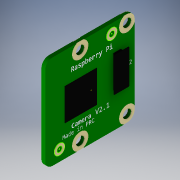
# Autodesk Inventor part: PicameraPCB
Saved by Autodesk Inventor 2022 (Build 260153000, 153)
## iProperties
Created: 2018-02-01
Part Number: PicameraPCB
Material: Genérico
Document SubType Name: Modeling
Designer: RafaX
Density: 1 g/cm^3
Appearance: Valor por defecto
Author: RafaX
Autodesk Inventor part; units mm, degrees
(part 1 of 2)
sketch "Boceto1" plane through (0, 0, 0) normal (0, 0, 1) x (1, 0, 0)
  line L0 (-9.7561, 12.3858) -> (10.1059, 12.3858)
  line L1 (12.1059, 10.3858) -> (12.1059, -10.6142)
  line L2 (10.1059, -12.6142) -> (-9.7561, -12.6142)
  line L3 (-11.7561, -10.6142) -> (-11.7561, 10.3858)
  arc A0 (-11.7561, -10.6142) -> (-9.7561, -12.6142) centre (-9.7561, -10.6142) ccw
  arc A1 (10.1059, -12.6142) -> (12.1059, -10.6142) centre (10.1059, -10.6142) ccw
  arc A2 (12.1059, 10.3858) -> (10.1059, 12.3858) centre (10.1059, 10.3858) ccw
  arc A3 (-9.7561, 12.3858) -> (-11.7561, 10.3858) centre (-9.7561, 10.3858) ccw
  point P0 (0, 0)
  point P1 (-11.7561, 12.3858)
  point P2 (12.1059, -12.6142)
  point P3 (12.1059, 12.3858)
  point P4 (-11.7561, -12.6142)
  point P5 (-9.7561, -10.6142)
  point P6 (2.7439, -10.6142)
  point P7 (-9.7561, 10.3858)
  point P8 (2.7439, 10.3858)
  dimension "d0" = 23.862
  dimension "d1" = 25
  dimension "d7" = 2
  dimension "d8" = 2
  dimension "d11" = 12.5
  dimension "d14" = 21
  dimension "d26" = 2
  constraints: 8 end point, 8 point on circle, 8 point on line, 8 tangent, 4 centre point, 3 equal radius, 2 horizontal, 2 parallel, 1 perpendicular, 1 vertical, 3 other
  measures "d0" distance of point (-11.756, 12.386) point (12.106, 12.386)
  measures "d1" distance of point (12.106, 12.386) point (12.106, -12.614)
  measures "d7" distance from line of L2 point (-9.756, -10.614)
  measures "d8" distance from line of L3 point (-9.756, -10.614)
  measures "d11" distance of point (-9.756, -10.614) point (2.744, -10.614)
  measures "d14" distance of point (-9.756, -10.614) point (-9.756, 10.386)
  measures "d26" radius of A0
extrude "PCB_EXT" add sketch "Boceto1" along normal blind 1
hole "PADS_PCB_DRILL" at (-9.7561, -10.6142, 0) at (2.7439, -10.6142, 0) at (-9.7561, 10.3858, 0) at (2.7439, 10.3858, 0) direction (0, 0, 1) diameter 2.2 end through all counterbore diameter 4.4 counterbore depth 0.12
sketch "Boceto2" plane through (0, 0, 1) normal (0, 0, 1) x (1, 0, 0)
  circle A0 centre (2.7468, 10.3904) radius 2.2
  circle A1 centre (2.7468, -10.6245) radius 2.2
  circle A2 centre (-9.7649, 10.3904) radius 2.2
  circle A3 centre (-9.7649, -10.6245) radius 2.2
  point P0 (0, 0)
  point P1 (2.7439, 10.3858)
  dimension "d27" = 4.4
  dimension "d28" = 4.4
  dimension "d29" = 4.4
  dimension "d30" = 4.4
  constraints: 4 centre point
  measures "d27" diameter of A0
  measures "d28" diameter of A1
  measures "d29" diameter of A2
  measures "d30" diameter of A3
extrude "PADS_PCB_DRILL_EXT" cut sketch "Boceto2" against normal blind 0.13
sketch "FOTO" plane through (0, 0, 1) normal (0, 0, 1) x (1, 0, 0)
  line L0 (-11.6696, 12.3223) -> (12.1528, 12.3223) construction
  line L1 (12.1528, 12.3223) -> (12.1528, -12.4777) construction
  line L2 (12.1528, -12.4777) -> (-11.6696, -12.4777) construction
  line L3 (-11.6696, -12.4777) -> (-11.6696, 12.3223) construction
  point P0 (0, 0)
  dimension "d57" = 24.8
  constraints: 2 other
  measures "d57" distance of L0.end L1.end
ref_plane "SUPERIOR_PADS" through (6.4264, 12.3858, 0.87) normal (0, 0, 1) x (1, 0, 0)
sketch "Boceto4" plane through (6.4264, 12.3858, 0.87) normal (0, 0, 1) x (1, 0, 0)
  arc A0 (-15.2525, -25) -> (-18.1824, -22.0747) centre (-16.1913, -23.0104) ccw projected
  arc A1 (-18.1824, -2.9311) -> (-15.2649, 0) centre (-16.1913, -1.9954) ccw projected
  arc A2 (-4.606, 0) -> (-2.7532, 0) centre (-3.6796, -1.9954) ccw projected
  circle A3 centre (-16.1824, -23) radius 1.1 projected
  circle A4 centre (-3.6824, -23) radius 1.1 projected
  line L0 (-18.1824, -2.9311) -> (-18.1824, -2) projected
  arc A5 (-16.1824, 0) -> (-18.1824, -2) centre (-16.1824, -2) ccw projected
  line L1 (-16.1824, 0) -> (-15.2649, 0) projected
  arc A6 (-16.1824, 0) -> (-18.1824, -2) centre (-16.1824, -2) ccw projected
  line L2 (-18.1824, -2.9311) -> (-18.1824, -2) projected
  arc A7 (-18.1824, -2.9311) -> (-15.2649, 0) centre (-16.1913, -1.9954) ccw projected
  circle A8 centre (-16.1824, -2) radius 1.1 projected
  line L3 (-4.606, 0) -> (-2.7532, 0) projected
  line L4 (-2.7408, -25) -> (-4.6184, -25) projected
  line L5 (-15.2525, -25) -> (-16.1824, -25) projected
  arc A9 (-18.1824, -23) -> (-16.1824, -25) centre (-16.1824, -23) ccw projected
  line L6 (-18.1824, -23) -> (-18.1824, -22.0747) projected
  circle A10 centre (-3.6824, -2) radius 1.1 projected
  arc A11 (-2.7408, -25) -> (-4.6184, -25) centre (-3.6796, -23.0104) ccw projected
  point P0 (-6.4264, -12.3858)
extrude "PADS_GOLDEN_UPPER_EXT" add sketch "Boceto4" along normal blind 0.07 separate body
ref_plane "INFERIOR_PADS" through (-3.5061, -12.6142, 0.12) normal (0, 0, -1) x (1, 0, 0)
sketch "Boceto5" plane through (-3.5061, -12.6142, 0.12) normal (0, 0, -1) x (1, 0, 0)
  line L0 (-6.25, 0) -> (-5.3335, 0) projected
  arc A0 (-6.25, 0) -> (-8.25, -2) centre (-6.25, -2) ccw projected
  line L1 (-8.25, -2.9165) -> (-8.25, -2) projected
  arc A1 (-8.25, -2.9165) -> (-5.3335, 0) centre (-6.25, -2) ccw projected
  circle A2 centre (-6.25, -2) radius 1.1 projected
  line L2 (5.3335, 0) -> (7.1665, 0) projected
  arc A3 (5.3335, 0) -> (7.1665, 0) centre (6.25, -2) ccw projected
  circle A4 centre (6.25, -2) radius 1.1 projected
  line L3 (7.1665, -25) -> (5.3335, -25) projected
  arc A5 (7.1665, -25) -> (5.3335, -25) centre (6.25, -23) ccw projected
  circle A6 centre (6.25, -23) radius 1.1 projected
  circle A7 centre (-6.25, -23) radius 1.1 projected
  line L4 (-5.3335, -25) -> (-6.25, -25) projected
  arc A8 (-5.3335, -25) -> (-8.25, -22.0835) centre (-6.25, -23) ccw projected
  line L5 (-8.25, -23) -> (-8.25, -22.0835) projected
  arc A9 (-8.25, -23) -> (-6.25, -25) centre (-6.25, -23) ccw projected
  point P0 (3.5061, -12.6142)
extrude "PADS_GOLDEN_LOWER_EXT" add sketch "Boceto5" along normal blind 0.07 separate body
sketch "text_front" plane through (0, 0, 1) normal (0, 0, 1) x (1, 0, 0)
  line L0 (5.2786, -8.033) -> (-7.7766, -8.033) construction
  line L1 (-7.7766, -8.033) -> (-7.7766, -6.6244) construction
  line L2 (-7.7766, -6.6244) -> (5.2786, -6.6244) construction
  line L3 (5.2786, -6.6244) -> (5.2786, -8.033) construction
  line L4 (-9.4094, -1.7368) -> (-11.3059, -1.7368) construction
  line L5 (-11.3059, -1.7368) -> (-11.3059, -0.6092) construction
  line L6 (-11.3059, -0.6092) -> (-9.4094, -0.6092) construction
  line L7 (-9.4094, -0.6092) -> (-9.4094, -1.7368) construction
  line L8 (5.1279, 5.2449) -> (-0.7022, 5.2449) construction
  line L9 (-0.7022, 5.2449) -> (-0.7022, 6.6125) construction
  line L10 (-0.7022, 6.6125) -> (5.1279, 6.6125) construction
  line L11 (5.1279, 6.6125) -> (5.1279, 5.2449) construction
  line L12 (-1.2173, 5.1295) -> (-5.0625, 5.1295) construction
  line L13 (-5.0625, 5.1295) -> (-5.0625, 6.3628) construction
  line L14 (-5.0625, 6.3628) -> (-1.2173, 6.3628) construction
  line L15 (-1.2173, 6.3628) -> (-1.2173, 5.1295) construction
  line L16 (7.5273, 6.703) -> (-2.1657, 6.703) construction
  line L17 (-2.1657, 6.703) -> (-2.1657, 7.9173) construction
  line L18 (-2.1657, 7.9173) -> (7.5273, 7.9173) construction
  line L19 (7.5273, 7.9173) -> (7.5273, 6.703) construction
  line L20 (4.6281, -6.6975) -> (4.7797, -7.0835)
  spline S0 degree 2 poles (4.7797, -7.0835) (4.8012, -7.1384) (4.8775, -7.1943) (4.9302, -7.1943) knots 0 0 0 1 2 2 2
  line L21 (4.9302, -7.1943) -> (4.9689, -7.1943)
  line L22 (4.9689, -7.1943) -> (4.9689, -6.6975)
  line L23 (4.9689, -6.6975) -> (5.1721, -6.6975)
  line L24 (5.1721, -6.6975) -> (5.1721, -7.8975)
  line L25 (5.1721, -7.8975) -> (4.8571, -7.8975)
  spline S1 degree 2 poles (4.8571, -7.8975) (4.7678, -7.8975) (4.6227, -7.8642) (4.5205, -7.7846) (4.4646, -7.6577) (4.4646, -7.5663) knots 0 0 0 1 2 3 4 4 4
  spline S2 degree 2 poles (4.4646, -7.5663) (4.4646, -7.4997) (4.5001, -7.3975) (4.5625, -7.3233) (4.6496, -7.2771) (4.7001, -7.2674) knots 0 0 0 1 2 3 4 4 4
  spline S3 degree 2 poles (4.7001, -7.2674) (4.6603, -7.2588) (4.5947, -7.1771) (4.5614, -7.0997) knots 0 0 0 1 2 2 2
  line L26 (4.5614, -7.0997) -> (4.3893, -6.6975)
  line L27 (4.3893, -6.6975) -> (4.6281, -6.6975)
  spline S4 degree 2 poles (4.6786, -7.5438) (4.6786, -7.6319) (4.7786, -7.7093) (4.8797, -7.7093) knots 0 0 0 1 2 2 2
  line L28 (4.8797, -7.7093) -> (4.9689, -7.7093)
  line L29 (4.9689, -7.7093) -> (4.9689, -7.3706)
  line L30 (4.9689, -7.3706) -> (4.8861, -7.3706)
  spline S5 degree 2 poles (4.8861, -7.3706) (4.8388, -7.3706) (4.7625, -7.3921) (4.7076, -7.4362) (4.6786, -7.5018) (4.6786, -7.5438) knots 0 0 0 1 2 3 4 4 4
  line L31 (3.7076, -6.6975) -> (3.713, -6.8201)
  spline S6 degree 2 poles (3.713, -6.8201) (3.7388, -6.7889) (3.7969, -6.7362) (3.8657, -6.6975) (3.9474, -6.676) (3.9969, -6.676) knots 0 0 0 1 2 3 4 4 4
  spline S7 degree 2 poles (3.9969, -6.676) (4.0614, -6.676) (4.1582, -6.719) (4.2248, -6.7943) (4.2582, -6.9007) (4.2582, -6.9653) knots 0 0 0 1 2 3 4 4 4
  spline S8 degree 2 poles (4.2582, -6.9653) (4.2582, -7.0308) (4.2076, -7.1427) (4.1044, -7.2233) (3.9506, -7.2696) (3.8463, -7.2696) knots 0 0 0 1 2 3 4 4 4
  line L32 (3.8463, -7.2696) -> (3.7367, -7.2696)
  line L33 (3.7367, -7.2696) -> (3.7367, -7.3255)
  spline S9 degree 2 poles (3.7367, -7.3255) (3.7367, -7.361) (3.7549, -7.419) (3.7947, -7.4599) (3.8592, -7.4814) (3.9066, -7.4814) knots 0 0 0 1 2 3 4 4 4
  spline S10 degree 2 poles (3.9066, -7.4814) (3.9807, -7.4814) (4.1259, -7.4438) (4.1936, -7.4104) knots 0 0 0 1 2 2 2
  line L34 (4.1936, -7.4104) -> (4.1936, -7.5889)
  spline S11 degree 2 poles (4.1936, -7.5889) (4.1334, -7.6158) (3.9754, -7.6502) (3.8904, -7.6502) knots 0 0 0 1 2 2 2
  spline S12 degree 2 poles (3.8904, -7.6502) (3.7969, -7.6502) (3.6625, -7.6115) (3.5764, -7.5319) (3.5345, -7.4136) (3.5345, -7.3351) knots 0 0 0 1 2 3 4 4 4
  line L35 (3.5345, -7.3351) -> (3.5345, -6.6975)
  line L36 (3.5345, -6.6975) -> (3.7076, -6.6975)
  line L37 (3.7367, -7.1093) -> (3.8592, -7.1093)
  spline S13 degree 2 poles (3.8592, -7.1093) (3.9109, -7.1093) (3.9818, -7.0878) (4.0259, -7.0491) (4.0474, -6.9986) (4.0474, -6.9706) knots 0 0 0 1 2 3 4 4 4
  spline S14 degree 2 poles (4.0474, -6.9706) (4.0474, -6.9136) (3.9807, -6.8534) (3.9238, -6.8534) knots 0 0 0 1 2 2 2
  spline S15 degree 2 poles (3.9238, -6.8534) (3.8818, -6.8534) (3.7915, -6.9212) (3.7367, -6.9846) knots 0 0 0 1 2 2 2
  line L38 (3.7367, -6.9846) -> (3.7367, -7.1093)
  spline S16 degree 2 poles (2.6119, -6.9717) (2.6119, -6.8921) (2.6754, -6.7792) (2.7797, -6.7083) (2.913, -6.676) (2.9818, -6.676) knots 0 0 0 1 2 3 4 4 4
  spline S17 degree 2 poles (2.9818, -6.676) (3.0743, -6.676) (3.2238, -6.6954) (3.2893, -6.7136) knots 0 0 0 1 2 2 2
  line L39 (3.2893, -6.7136) -> (3.2893, -6.9158)
  spline S18 degree 2 poles (3.2893, -6.9158) (3.2119, -6.8803) (3.0571, -6.8481) (2.9893, -6.8481) knots 0 0 0 1 2 2 2
  spline S19 degree 2 poles (2.9893, -6.8481) (2.9098, -6.8481) (2.8313, -6.904) (2.8313, -6.9491) knots 0 0 0 1 2 2 2
  spline S20 degree 2 poles (2.8313, -6.9491) (2.8313, -6.9706) (2.8474, -7.005) (2.8936, -7.0373) (2.9754, -7.0717) (3.0431, -7.0921) knots 0 0 0 1 2 3 4 4 4
  spline S21 degree 2 poles (3.0431, -7.0921) (3.1044, -7.1115) (3.1979, -7.1599) (3.2592, -7.2265) (3.2893, -7.3136) (3.2893, -7.3728) knots 0 0 0 1 2 3 4 4 4
  spline S22 degree 2 poles (3.2893, -7.3728) (3.2893, -7.4298) (3.2431, -7.5308) (3.1517, -7.6061) (3.0141, -7.6502) (2.9227, -7.6502) knots 0 0 0 1 2 3 4 4 4
  spline S23 degree 2 poles (2.9227, -7.6502) (2.8431, -7.6502) (2.7216, -7.6319) (2.6743, -7.6212) knots 0 0 0 1 2 2 2
  line L40 (2.6743, -7.6212) -> (2.6743, -7.4384)
  spline S24 degree 2 poles (2.6743, -7.4384) (2.7463, -7.4642) (2.8721, -7.4857) (2.9345, -7.4857) knots 0 0 0 1 2 2 2
  spline S25 degree 2 poles (2.9345, -7.4857) (2.9969, -7.4857) (3.0711, -7.4362) (3.0711, -7.3921) knots 0 0 0 1 2 2 2
  spline S26 degree 2 poles (3.0711, -7.3921) (3.0711, -7.3706) (3.0571, -7.3373) (3.013, -7.3061) (2.9345, -7.2728) (2.87, -7.2524) knots 0 0 0 1 2 3 4 4 4
  spline S27 degree 2 poles (2.87, -7.2524) (2.7969, -7.2287) (2.6979, -7.1771) (2.6377, -7.1104) (2.6119, -7.0265) (2.6119, -6.9717) knots 0 0 0 1 2 3 4 4 4
  spline S28 degree 2 poles (1.6184, -7.1803) (1.6184, -7.0524) (1.684, -6.8642) (1.8001, -6.7405) (1.9592, -6.6814) (2.0517, -6.6814) knots 0 0 0 1 2 3 4 4 4
  spline S29 degree 2 poles (2.0517, -6.6814) (2.084, -6.6814) (2.1463, -6.69) (2.1721, -6.6975) knots 0 0 0 1 2 2 2
  line L41 (2.1721, -6.6975) -> (2.1721, -6.333)
  line L42 (2.1721, -6.333) -> (2.3732, -6.333)
  line L43 (2.3732, -6.333) -> (2.3732, -7.6308)
  line L44 (2.3732, -7.6308) -> (2.199, -7.6308)
  line L45 (2.199, -7.6308) -> (2.1947, -7.4932)
  spline S30 degree 2 poles (2.1947, -7.4932) (2.1689, -7.5287) (2.113, -7.5878) (2.0485, -7.6287) (1.9743, -7.6502) (1.9281, -7.6502) knots 0 0 0 1 2 3 4 4 4
  spline S31 degree 2 poles (1.9281, -7.6502) (1.8539, -7.6502) (1.7388, -7.5846) (1.6603, -7.462) (1.6184, -7.2889) (1.6184, -7.1803) knots 0 0 0 1 2 3 4 4 4
  spline S32 degree 2 poles (1.8302, -7.1717) (1.8302, -7.2481) (1.8496, -7.3567) (1.8872, -7.4265) (1.941, -7.4588) (1.9754, -7.4588) knots 0 0 0 1 2 3 4 4 4
  spline S33 degree 2 poles (1.9754, -7.4588) (2.027, -7.4588) (2.1195, -7.3674) (2.1721, -7.2878) knots 0 0 0 1 2 2 2
  line L46 (2.1721, -7.2878) -> (2.1721, -6.8803)
  spline S34 degree 2 poles (2.1721, -6.8803) (2.1485, -6.8706) (2.0775, -6.8577) (2.041, -6.8577) knots 0 0 0 1 2 2 2
  spline S35 degree 2 poles (2.041, -6.8577) (1.9936, -6.8577) (1.9152, -6.9018) (1.8592, -6.9825) (1.8302, -7.0986) (1.8302, -7.1717) knots 0 0 0 1 2 3 4 4 4
  spline S36 degree 2 poles (0.6883, -7.1803) (0.6883, -7.0524) (0.7539, -6.8642) (0.87, -6.7405) (1.0291, -6.6814) (1.1216, -6.6814) knots 0 0 0 1 2 3 4 4 4
  spline S37 degree 2 poles (1.1216, -6.6814) (1.2141, -6.6814) (1.3711, -6.7115) (1.4431, -6.7373) knots 0 0 0 1 2 2 2
  line L47 (1.4431, -6.7373) -> (1.4431, -7.9954)
  line L48 (1.4431, -7.9954) -> (1.242, -7.9954)
  line L49 (1.242, -7.9954) -> (1.242, -7.69)
  line L50 (1.242, -7.69) -> (1.2506, -7.5061)
  spline S38 degree 2 poles (1.2506, -7.5061) (1.2044, -7.5717) (1.0829, -7.6502) (0.9979, -7.6502) knots 0 0 0 1 2 2 2
  spline S39 degree 2 poles (0.9979, -7.6502) (0.9238, -7.6502) (0.8087, -7.5846) (0.7302, -7.462) (0.6883, -7.2889) (0.6883, -7.1803) knots 0 0 0 1 2 3 4 4 4
  spline S40 degree 2 poles (0.9001, -7.1717) (0.9001, -7.2481) (0.9195, -7.3567) (0.9571, -7.4265) (1.0109, -7.4588) (1.0453, -7.4588) knots 0 0 0 1 2 3 4 4 4
  spline S41 degree 2 poles (1.0453, -7.4588) (1.0969, -7.4588) (1.1893, -7.3674) (1.242, -7.2878) knots 0 0 0 1 2 2 2
  line L51 (1.242, -7.2878) -> (1.242, -6.8803)
  spline S42 degree 2 poles (1.242, -6.8803) (1.2184, -6.8706) (1.1474, -6.8577) (1.1109, -6.8577) knots 0 0 0 1 2 2 2
  spline S43 degree 2 poles (1.1109, -6.8577) (1.0635, -6.8577) (0.985, -6.9018) (0.9291, -6.9825) (0.9001, -7.0986) (0.9001, -7.1717) knots 0 0 0 1 2 3 4 4 4
  spline S44 degree 2 poles (-0.2182, -7.2351) (-0.2182, -7.2126) (-0.215, -7.1394) (-0.2128, -7.1072) knots 0 0 0 1 2 2 2
  line L52 (-0.2128, -7.1072) -> (0.3388, -7.1072)
  spline S45 degree 2 poles (0.3388, -7.1072) (0.3388, -7.0459) (0.3055, -6.9524) (0.2431, -6.8889) (0.156, -6.8556) (0.1033, -6.8556) knots 0 0 0 1 2 3 4 4 4
  spline S46 degree 2 poles (0.1033, -6.8556) (0.042, -6.8556) (-0.0967, -6.8771) (-0.1719, -6.9007) knots 0 0 0 1 2 2 2
  line L53 (-0.1719, -6.9007) -> (-0.1719, -6.7222)
  spline S47 degree 2 poles (-0.1719, -6.7222) (-0.1397, -6.7126) (-0.0644, -6.6954) (0.0152, -6.6825) (0.0958, -6.676) (0.1345, -6.676) knots 0 0 0 1 2 3 4 4 4
  spline S48 degree 2 poles (0.1345, -6.676) (0.2302, -6.676) (0.3818, -6.7373) (0.4872, -6.8556) (0.5442, -7.0298) (0.5442, -7.1448) knots 0 0 0 1 2 3 4 4 4
  spline S49 degree 2 poles (0.5442, -7.1448) (0.5442, -7.2588) (0.4872, -7.4448) (0.385, -7.5782) (0.2388, -7.6502) (0.1496, -7.6502) knots 0 0 0 1 2 3 4 4 4
  spline S50 degree 2 poles (0.1496, -7.6502) (0.0603, -7.6502) (-0.0773, -7.5889) (-0.1698, -7.4792) (-0.2182, -7.3265) (-0.2182, -7.2351) knots 0 0 0 1 2 3 4 4 4
  spline S51 degree 2 poles (-0.0128, -7.2674) (-0.0139, -7.3233) (0.013, -7.405) (0.0582, -7.4577) (0.1184, -7.4835) (0.1528, -7.4835) knots 0 0 0 1 2 3 4 4 4
  spline S52 degree 2 poles (0.1528, -7.4835) (0.2291, -7.4835) (0.327, -7.3706) (0.3356, -7.2674) knots 0 0 0 1 2 2 2
  line L54 (0.3356, -7.2674) -> (-0.0128, -7.2674)
  spline S53 degree 2 poles (-0.9569, -7.2674) (-0.959, -7.3201) (-0.9461, -7.3932) (-0.9193, -7.4416) (-0.8795, -7.4631) (-0.8537, -7.4631) knots 0 0 0 1 2 3 4 4 4
  spline S54 degree 2 poles (-0.8537, -7.4631) (-0.8096, -7.4631) (-0.7139, -7.3814) (-0.6569, -7.2878) knots 0 0 0 1 2 2 2
  line L55 (-0.6569, -7.2878) -> (-0.6569, -6.6975)
  line L56 (-0.6569, -6.6975) -> (-0.4504, -6.6975)
  line L57 (-0.4504, -6.6975) -> (-0.4504, -7.6308)
  line L58 (-0.4504, -7.6308) -> (-0.6332, -7.6308)
  line L59 (-0.6332, -7.6308) -> (-0.6408, -7.4943)
  spline S55 degree 2 poles (-0.6408, -7.4943) (-0.6612, -7.5308) (-0.7139, -7.5878) (-0.7773, -7.6287) (-0.8547, -7.6502) (-0.901, -7.6502) knots 0 0 0 1 2 3 4 4 4
  spline S56 degree 2 poles (-0.901, -7.6502) (-0.9644, -7.6502) (-1.0623, -7.6018) (-1.13, -7.5061) (-1.1623, -7.362) (-1.159, -7.2674) knots 0 0 0 1 2 3 4 4 4
  line L60 (-1.159, -7.2674) -> (-0.9569, -7.2674)
  spline S57 degree 2 poles (-1.887, -7.2674) (-1.8891, -7.3201) (-1.8762, -7.3932) (-1.8494, -7.4416) (-1.8096, -7.4631) (-1.7838, -7.4631) knots 0 0 0 1 2 3 4 4 4
  spline S58 degree 2 poles (-1.7838, -7.4631) (-1.7397, -7.4631) (-1.644, -7.3814) (-1.587, -7.2878) knots 0 0 0 1 2 2 2
  line L61 (-1.587, -7.2878) -> (-1.587, -6.6975)
  line L62 (-1.587, -6.6975) -> (-1.3805, -6.6975)
  line L63 (-1.3805, -6.6975) -> (-1.3805, -7.6308)
  line L64 (-1.3805, -7.6308) -> (-1.5633, -7.6308)
  line L65 (-1.5633, -7.6308) -> (-1.5709, -7.4943)
  spline S59 degree 2 poles (-1.5709, -7.4943) (-1.5913, -7.5308) (-1.644, -7.5878) (-1.7074, -7.6287) (-1.7848, -7.6502) (-1.8311, -7.6502) knots 0 0 0 1 2 3 4 4 4
  spline S60 degree 2 poles (-1.8311, -7.6502) (-1.8945, -7.6502) (-1.9924, -7.6018) (-2.0601, -7.5061) (-2.0924, -7.362) (-2.0891, -7.2674) knots 0 0 0 1 2 3 4 4 4
  line L66 (-2.0891, -7.2674) -> (-1.887, -7.2674)
  spline S61 degree 2 poles (-2.7816, -6.7997) (-2.7375, -6.6782) (-2.6429, -6.4954) (-2.5289, -6.3739) (-2.3891, -6.3115) (-2.3031, -6.3115) knots 0 0 0 1 2 3 4 4 4
  spline S62 degree 2 poles (-2.3031, -6.3115) (-2.2816, -6.3115) (-2.2332, -6.3169) (-2.2074, -6.3212) knots 0 0 0 1 2 2 2
  line L67 (-2.2074, -6.3212) -> (-2.2074, -6.5115)
  spline S63 degree 2 poles (-2.2074, -6.5115) (-2.2171, -6.5093) (-2.2429, -6.505) (-2.2709, -6.5018) (-2.2999, -6.4997) (-2.3128, -6.4997) knots 0 0 0 1 2 3 4 4 4
  spline S64 degree 2 poles (-2.3128, -6.4997) (-2.3472, -6.4997) (-2.4064, -6.5298) (-2.4569, -6.5814) (-2.4988, -6.6545) (-2.5139, -6.6975) knots 0 0 0 1 2 3 4 4 4
  line L68 (-2.5139, -6.6975) -> (-2.1816, -7.6308)
  line L69 (-2.1816, -7.6308) -> (-2.4064, -7.6308)
  line L70 (-2.4064, -7.6308) -> (-2.5805, -7.1018)
  line L71 (-2.5805, -7.1018) -> (-2.6322, -6.9308)
  line L72 (-2.6322, -6.9308) -> (-2.6838, -7.0943)
  line L73 (-2.6838, -7.0943) -> (-2.859, -7.6308)
  line L74 (-2.859, -7.6308) -> (-3.0752, -7.6308)
  line L75 (-3.0752, -7.6308) -> (-2.7816, -6.7997)
  spline S65 degree 2 poles (-4.8827, -7.5158) (-4.8827, -7.4222) (-4.8268, -7.2631) (-4.716, -7.147) (-4.5515, -7.0835) (-4.4418, -7.0835) knots 0 0 0 1 2 3 4 4 4
  line L76 (-4.4418, -7.0835) -> (-4.3386, -7.0835)
  line L77 (-4.3386, -7.0835) -> (-4.3386, -6.6975)
  line L78 (-4.3386, -6.6975) -> (-4.1343, -6.6975)
  line L79 (-4.1343, -6.6975) -> (-4.1343, -7.8975)
  line L80 (-4.1343, -7.8975) -> (-4.4504, -7.8975)
  spline S66 degree 2 poles (-4.4504, -7.8975) (-4.5547, -7.8975) (-4.716, -7.847) (-4.8257, -7.7502) (-4.8827, -7.6072) (-4.8827, -7.5158) knots 0 0 0 1 2 3 4 4 4
  spline S67 degree 2 poles (-4.6698, -7.4997) (-4.6698, -7.5481) (-4.6429, -7.6255) (-4.587, -7.6814) (-4.5031, -7.7104) (-4.4451, -7.7104) knots 0 0 0 1 2 3 4 4 4
  line L81 (-4.4451, -7.7104) -> (-4.3386, -7.7104)
  line L82 (-4.3386, -7.7104) -> (-4.3386, -7.2706)
  line L83 (-4.3386, -7.2706) -> (-4.4515, -7.2706)
  spline S68 degree 2 poles (-4.4515, -7.2706) (-4.5053, -7.2706) (-4.5859, -7.3029) (-4.6408, -7.3631) (-4.6698, -7.4481) (-4.6698, -7.4997) knots 0 0 0 1 2 3 4 4 4
  line L84 (-5.3386, -7.4556) -> (-5.101, -7.4556)
  line L85 (-5.101, -7.4556) -> (-5.101, -7.6308)
  line L86 (-5.101, -7.6308) -> (-5.5451, -7.6308)
  line L87 (-5.5451, -7.6308) -> (-5.5451, -6.8717)
  line L88 (-5.5451, -6.8717) -> (-5.787, -6.8717)
  line L89 (-5.787, -6.8717) -> (-5.787, -6.6975)
  line L90 (-5.787, -6.6975) -> (-5.0719, -6.6975)
  line L91 (-5.0719, -6.6975) -> (-5.0719, -6.8717)
  line L92 (-5.0719, -6.8717) -> (-5.3386, -6.8717)
  line L93 (-5.3386, -6.8717) -> (-5.3386, -7.4556)
  spline S69 degree 2 poles (-5.5612, -7.8857) (-5.5612, -7.8556) (-5.5418, -7.8018) (-5.5064, -7.7631) (-5.458, -7.7394) (-5.43, -7.7394) knots 0 0 0 1 2 3 4 4 4
  spline S70 degree 2 poles (-5.43, -7.7394) (-5.4021, -7.7394) (-5.3537, -7.7631) (-5.3171, -7.8018) (-5.2977, -7.8556) (-5.2977, -7.8857) knots 0 0 0 1 2 3 4 4 4
  spline S71 degree 2 poles (-5.2977, -7.8857) (-5.2977, -7.9158) (-5.3171, -7.9696) (-5.3537, -8.0093) (-5.4021, -8.033) (-5.43, -8.033) knots 0 0 0 1 2 3 4 4 4
  spline S72 degree 2 poles (-5.43, -8.033) (-5.458, -8.033) (-5.5064, -8.0093) (-5.5418, -7.9696) (-5.5612, -7.9158) (-5.5612, -7.8857) knots 0 0 0 1 2 3 4 4 4
  line L94 (-10.0331, -1.7225) -> (-10.0331, -1.028)
  spline S73 degree 2 poles (-10.0331, -1.028) (-10.0331, -0.9635) (-9.9982, -0.8479) (-9.9256, -0.7619) (-9.8154, -0.7117) (-9.7419, -0.7117) knots 0 0 0 1 2 3 4 4 4
  spline S74 degree 2 poles (-9.7419, -0.7117) (-9.7141, -0.7117) (-9.6568, -0.7198) (-9.603, -0.735) (-9.5564, -0.7556) (-9.5394, -0.7673) knots 0 0 0 1 2 3 4 4 4
  line L95 (-9.5394, -0.7673) -> (-9.5394, -0.9044)
  spline S75 degree 2 poles (-9.5394, -0.9044) (-9.5833, -0.8703) (-9.6908, -0.83) (-9.7428, -0.83) knots 0 0 0 1 2 2 2
  spline S76 degree 2 poles (-9.7428, -0.83) (-9.8207, -0.83) (-9.905, -0.9321) (-9.905, -1.028) knots 0 0 0 1 2 2 2
  line L96 (-9.905, -1.028) -> (-9.905, -1.6051)
  line L97 (-9.905, -1.6051) -> (-9.551, -1.6051)
  line L98 (-9.551, -1.6051) -> (-9.551, -1.7225)
  line L99 (-9.551, -1.7225) -> (-10.0331, -1.7225)
  line L100 (-10.9274, -0.7225) -> (-10.3154, -0.7225)
  line L101 (-10.3154, -0.7225) -> (-10.3154, -0.8416)
  line L102 (-10.3154, -0.8416) -> (-10.5555, -1.0988)
  spline S77 degree 2 poles (-10.5555, -1.0988) (-10.6146, -1.1615) (-10.689, -1.2538) (-10.7302, -1.3291) (-10.7437, -1.3963) (-10.7437, -1.4357) knots 0 0 0 1 2 3 4 4 4
  spline S78 degree 2 poles (-10.7437, -1.4357) (-10.7437, -1.4725) (-10.7258, -1.5388) (-10.6872, -1.5898) (-10.6263, -1.6185) (-10.5833, -1.6185) knots 0 0 0 1 2 3 4 4 4
  spline S79 degree 2 poles (-10.5833, -1.6185) (-10.5241, -1.6185) (-10.4274, -1.5621) (-10.387, -1.5164) knots 0 0 0 1 2 2 2
  line L103 (-10.387, -1.5164) -> (-10.3189, -1.6051)
  spline S80 degree 2 poles (-10.3189, -1.6051) (-10.3709, -1.6642) (-10.5089, -1.7368) (-10.5994, -1.7368) knots 0 0 0 1 2 2 2
  spline S81 degree 2 poles (-10.5994, -1.7368) (-10.6612, -1.7368) (-10.7634, -1.6965) (-10.8369, -1.6212) (-10.8781, -1.5128) (-10.8781, -1.4447) knots 0 0 0 1 2 3 4 4 4
  spline S82 degree 2 poles (-10.8781, -1.4447) (-10.8781, -1.3873) (-10.8494, -1.2897) (-10.7921, -1.192) (-10.7042, -1.0881) (-10.6442, -1.0262) knots 0 0 0 1 2 3 4 4 4
  line L104 (-10.6442, -1.0262) -> (-10.4758, -0.8497)
  line L105 (-10.4758, -0.8497) -> (-10.9274, -0.8497)
  line L106 (-10.9274, -0.8497) -> (-10.9274, -0.7225)
  line L107 (-2.1754, 5.1467) -> (-1.7958, 6.3467)
  line L108 (-1.7958, 6.3467) -> (-1.5915, 6.3467)
  line L109 (-1.5915, 6.3467) -> (-1.2205, 5.1467)
  line L110 (-1.2205, 5.1467) -> (-1.3926, 5.1467)
  line L111 (-1.3926, 5.1467) -> (-1.6334, 5.9553)
  line L112 (-1.6334, 5.9553) -> (-1.7012, 6.1929)
  line L113 (-1.7012, 6.1929) -> (-1.7711, 5.9553)
  line L114 (-1.7711, 5.9553) -> (-2.013, 5.1467)
  line L115 (-2.013, 5.1467) -> (-2.1754, 5.1467)
  line L116 (-3.0388, 6.3467) -> (-2.3044, 6.3467)
  line L117 (-2.3044, 6.3467) -> (-2.3044, 6.2037)
  line L118 (-2.3044, 6.2037) -> (-2.5926, 5.8951)
  spline S83 degree 2 poles (-2.5926, 5.8951) (-2.6635, 5.8198) (-2.7528, 5.7091) (-2.8023, 5.6187) (-2.8184, 5.5381) (-2.8184, 5.4908) knots 0 0 0 1 2 3 4 4 4
  spline S84 degree 2 poles (-2.8184, 5.4908) (-2.8184, 5.4467) (-2.7969, 5.3671) (-2.7506, 5.3058) (-2.6775, 5.2714) (-2.6259, 5.2714) knots 0 0 0 1 2 3 4 4 4
  spline S85 degree 2 poles (-2.6259, 5.2714) (-2.5549, 5.2714) (-2.4388, 5.3392) (-2.3904, 5.394) knots 0 0 0 1 2 2 2
  line L119 (-2.3904, 5.394) -> (-2.3087, 5.2876)
  spline S86 degree 2 poles (-2.3087, 5.2876) (-2.3711, 5.2166) (-2.5367, 5.1295) (-2.6453, 5.1295) knots 0 0 0 1 2 2 2
  spline S87 degree 2 poles (-2.6453, 5.1295) (-2.7195, 5.1295) (-2.842, 5.1779) (-2.9302, 5.2682) (-2.9797, 5.3983) (-2.9797, 5.48) knots 0 0 0 1 2 3 4 4 4
  spline S88 degree 2 poles (-2.9797, 5.48) (-2.9797, 5.5488) (-2.9453, 5.6661) (-2.8764, 5.7833) (-2.7711, 5.908) (-2.699, 5.9822) knots 0 0 0 1 2 3 4 4 4
  line L120 (-2.699, 5.9822) -> (-2.4969, 6.194)
  line L121 (-2.4969, 6.194) -> (-3.0388, 6.194)
  line L122 (-3.0388, 6.194) -> (-3.0388, 6.3467)
  spline S89 degree 2 poles (-3.6141, 6.0574) (-3.6431, 6.0574) (-3.6947, 6.0811) (-3.7334, 6.123) (-3.7549, 6.18) (-3.7549, 6.2112) knots 0 0 0 1 2 3 4 4 4
  spline S90 degree 2 poles (-3.7549, 6.2112) (-3.7549, 6.2424) (-3.7334, 6.2983) (-3.6947, 6.3392) (-3.6431, 6.3628) (-3.6141, 6.3628) knots 0 0 0 1 2 3 4 4 4
  spline S91 degree 2 poles (-3.6141, 6.3628) (-3.584, 6.3628) (-3.5324, 6.3392) (-3.4937, 6.2983) (-3.4721, 6.2424) (-3.4721, 6.2112) knots 0 0 0 1 2 3 4 4 4
  spline S92 degree 2 poles (-3.4721, 6.2112) (-3.4721, 6.18) (-3.4937, 6.123) (-3.5324, 6.0811) (-3.584, 6.0574) (-3.6141, 6.0574) knots 0 0 0 1 2 3 4 4 4
  line L123 (-4.9528, 6.3467) -> (-4.2517, 6.3467)
  line L124 (-4.2517, 6.3467) -> (-4.2517, 6.1983)
  line L125 (-4.2517, 6.1983) -> (-4.5388, 6.1983)
  line L126 (-4.5388, 6.1983) -> (-4.5388, 5.322)
  line L127 (-4.5388, 5.322) -> (-4.2711, 5.4779)
  line L128 (-4.2711, 5.4779) -> (-4.2162, 5.3424)
  line L129 (-4.2162, 5.3424) -> (-4.5711, 5.1413)
  line L130 (-4.5711, 5.1413) -> (-4.7033, 5.1413)
  line L131 (-4.7033, 5.1413) -> (-4.7033, 6.1983)
  line L132 (-4.7033, 6.1983) -> (-4.9528, 6.1983)
  line L133 (-4.9528, 6.1983) -> (-4.9528, 6.3467)
  spline S93 degree 2 poles (4.3424, 6.3173) (4.4104, 6.3469) (4.5375, 6.3755) (4.6065, 6.3755) knots 0 0 0 1 2 2 2
  spline S94 degree 2 poles (4.6065, 6.3755) (4.7169, 6.3755) (4.8864, 6.3055) (5.0037, 6.1675) (5.0639, 5.9635) (5.0639, 5.8274) knots 0 0 0 1 2 3 4 4 4
  spline S95 degree 2 poles (5.0639, 5.8274) (5.0639, 5.6885) (4.9978, 5.4726) (4.8756, 5.3238) (4.7011, 5.2449) (4.5927, 5.2449) knots 0 0 0 1 2 3 4 4 4
  spline S96 degree 2 poles (4.5927, 5.2449) (4.5572, 5.2449) (4.4951, 5.2488) (4.436, 5.2577) (4.3749, 5.2735) (4.3424, 5.2853) knots 0 0 0 1 2 3 4 4 4
  line L134 (4.3424, 5.2853) -> (4.3424, 5.4903)
  spline S97 degree 2 poles (4.3424, 5.4903) (4.4084, 5.4568) (4.5296, 5.4282) (4.5789, 5.4282) knots 0 0 0 1 2 2 2
  spline S98 degree 2 poles (4.5789, 5.4282) (4.6509, 5.4282) (4.7544, 5.4844) (4.8214, 5.5859) (4.8529, 5.7269) (4.8529, 5.8107) knots 0 0 0 1 2 3 4 4 4
  spline S99 degree 2 poles (4.8529, 5.8107) (4.8529, 5.9004) (4.8204, 6.0403) (4.7534, 6.1389) (4.6479, 6.1902) (4.576, 6.1902) knots 0 0 0 1 2 3 4 4 4
  spline S100 degree 2 poles (4.576, 6.1902) (4.5503, 6.1902) (4.4902, 6.1793) (4.4281, 6.1616) (4.368, 6.1369) (4.3424, 6.1241) knots 0 0 0 1 2 3 4 4 4
  line L135 (4.3424, 6.1241) -> (4.3424, 6.3173)
  line L136 (3.6396, 6.3607) -> (3.6445, 6.2483)
  spline S101 degree 2 poles (3.6445, 6.2483) (3.6692, 6.2769) (3.7244, 6.3252) (3.7894, 6.3607) (3.8673, 6.3804) (3.9136, 6.3804) knots 0 0 0 1 2 3 4 4 4
  spline S102 degree 2 poles (3.9136, 6.3804) (3.9747, 6.3804) (4.0664, 6.341) (4.1295, 6.272) (4.161, 6.1744) (4.161, 6.1152) knots 0 0 0 1 2 3 4 4 4
  spline S103 degree 2 poles (4.161, 6.1152) (4.161, 6.0551) (4.1137, 5.9526) (4.0161, 5.8787) (3.8692, 5.8363) (3.7707, 5.8363) knots 0 0 0 1 2 3 4 4 4
  line L137 (3.7707, 5.8363) -> (3.6672, 5.8363)
  line L138 (3.6672, 5.8363) -> (3.6672, 5.785)
  spline S104 degree 2 poles (3.6672, 5.785) (3.6672, 5.7525) (3.6839, 5.6993) (3.7224, 5.6618) (3.7835, 5.6421) (3.8278, 5.6421) knots 0 0 0 1 2 3 4 4 4
  spline S105 degree 2 poles (3.8278, 5.6421) (3.8988, 5.6421) (4.0358, 5.6766) (4.0999, 5.7072) knots 0 0 0 1 2 2 2
  line L139 (4.0999, 5.7072) -> (4.0999, 5.5436)
  spline S106 degree 2 poles (4.0999, 5.5436) (4.0427, 5.5189) (3.8929, 5.4874) (3.8121, 5.4874) knots 0 0 0 1 2 2 2
  spline S107 degree 2 poles (3.8121, 5.4874) (3.7244, 5.4874) (3.5972, 5.5229) (3.5154, 5.5958) (3.476, 5.7042) (3.476, 5.7762) knots 0 0 0 1 2 3 4 4 4
  line L140 (3.476, 5.7762) -> (3.476, 6.3607)
  line L141 (3.476, 6.3607) -> (3.6396, 6.3607)
  line L142 (3.6672, 5.9832) -> (3.7835, 5.9832)
  spline S108 degree 2 poles (3.7835, 5.9832) (3.8318, 5.9832) (3.8988, 6.0029) (3.9412, 6.0384) (3.9609, 6.0847) (3.9609, 6.1103) knots 0 0 0 1 2 3 4 4 4
  spline S109 degree 2 poles (3.9609, 6.1103) (3.9609, 6.1626) (3.8988, 6.2178) (3.8446, 6.2178) knots 0 0 0 1 2 2 2
  spline S110 degree 2 poles (3.8446, 6.2178) (3.8042, 6.2178) (3.7184, 6.1557) (3.6672, 6.0975) knots 0 0 0 1 2 2 2
  line L143 (3.6672, 6.0975) -> (3.6672, 5.9832)
  line L144 (2.6953, 6.3607) -> (2.6953, 5.7781)
  spline S111 degree 2 poles (2.6953, 5.7781) (2.6953, 5.7466) (2.6993, 5.6983) (2.7081, 5.6658) (2.7259, 5.65) (2.7416, 5.65) knots 0 0 0 1 2 3 4 4 4
  spline S112 degree 2 poles (2.7416, 5.65) (2.7663, 5.65) (2.8126, 5.721) (2.8432, 5.8057) knots 0 0 0 1 2 2 2
  line L145 (2.8432, 5.8057) -> (2.8432, 6.3607)
  line L146 (2.8432, 6.3607) -> (3.0068, 6.3607)
  line L147 (3.0068, 6.3607) -> (3.0068, 5.7781)
  spline S113 degree 2 poles (3.0068, 5.7781) (3.0068, 5.7466) (3.0097, 5.6983) (3.0186, 5.6658) (3.0373, 5.65) (3.0531, 5.65) knots 0 0 0 1 2 3 4 4 4
  spline S114 degree 2 poles (3.0531, 5.65) (3.0738, 5.65) (3.1241, 5.721) (3.1546, 5.8057) knots 0 0 0 1 2 2 2
  line L148 (3.1546, 5.8057) -> (3.1546, 6.3607)
  line L149 (3.1546, 6.3607) -> (3.3192, 6.3607)
  line L150 (3.3192, 6.3607) -> (3.3192, 5.5051)
  line L151 (3.3192, 5.5051) -> (3.1773, 5.5051)
  line L152 (3.1773, 5.5051) -> (3.1744, 5.6303)
  spline S115 degree 2 poles (3.1744, 5.6303) (3.1576, 5.5919) (3.1231, 5.5386) (3.0837, 5.5041) (3.0393, 5.4884) (3.0107, 5.4884) knots 0 0 0 1 2 3 4 4 4
  spline S116 degree 2 poles (3.0107, 5.4884) (2.9447, 5.4884) (2.8747, 5.5633) (2.8698, 5.6303) knots 0 0 0 1 2 2 2
  spline S117 degree 2 poles (2.8698, 5.6303) (2.8511, 5.5919) (2.8146, 5.5386) (2.7752, 5.5041) (2.7288, 5.4884) (2.7002, 5.4884) knots 0 0 0 1 2 3 4 4 4
  spline S118 degree 2 poles (2.7002, 5.4884) (2.6135, 5.4884) (2.5307, 5.6195) (2.5307, 5.7466) knots 0 0 0 1 2 2 2
  line L153 (2.5307, 5.7466) -> (2.5307, 6.3607)
  line L154 (2.5307, 6.3607) -> (2.6953, 6.3607)
  spline S119 degree 2 poles (1.683, 5.8678) (1.683, 5.8885) (1.685, 5.9556) (1.688, 5.9851) knots 0 0 0 1 2 2 2
  line L155 (1.688, 5.9851) -> (2.2104, 5.9851)
  spline S120 degree 2 poles (2.2104, 5.9851) (2.2104, 6.0413) (2.1788, 6.1271) (2.1197, 6.1852) (2.0379, 6.2158) (1.9876, 6.2158) knots 0 0 0 1 2 3 4 4 4
  spline S121 degree 2 poles (1.9876, 6.2158) (1.9295, 6.2158) (1.7974, 6.1961) (1.7264, 6.1744) knots 0 0 0 1 2 2 2
  line L156 (1.7264, 6.1744) -> (1.7264, 6.338)
  spline S122 degree 2 poles (1.7264, 6.338) (1.757, 6.3469) (1.8289, 6.3626) (1.9038, 6.3745) (1.9807, 6.3804) (2.0162, 6.3804) knots 0 0 0 1 2 3 4 4 4
  spline S123 degree 2 poles (2.0162, 6.3804) (2.1069, 6.3804) (2.2508, 6.3242) (2.3513, 6.2158) (2.4045, 6.0561) (2.4045, 5.9506) knots 0 0 0 1 2 3 4 4 4
  spline S124 degree 2 poles (2.4045, 5.9506) (2.4045, 5.8462) (2.3513, 5.6756) (2.2547, 5.5534) (2.1157, 5.4874) (2.031, 5.4874) knots 0 0 0 1 2 3 4 4 4
  spline S125 degree 2 poles (2.031, 5.4874) (1.9462, 5.4874) (1.8161, 5.5436) (1.7284, 5.6441) (1.683, 5.7841) (1.683, 5.8678) knots 0 0 0 1 2 3 4 4 4
  spline S126 degree 2 poles (1.8772, 5.8383) (1.8762, 5.787) (1.9019, 5.7121) (1.9442, 5.6638) (2.0014, 5.6402) (2.0339, 5.6402) knots 0 0 0 1 2 3 4 4 4
  spline S127 degree 2 poles (2.0339, 5.6402) (2.1069, 5.6402) (2.1985, 5.7436) (2.2074, 5.8383) knots 0 0 0 1 2 2 2
  line L157 (2.2074, 5.8383) -> (1.8772, 5.8383)
  spline S128 degree 2 poles (0.9822, 5.8383) (0.9813, 5.79) (0.9931, 5.7229) (1.0187, 5.6786) (1.0562, 5.6589) (1.0808, 5.6589) knots 0 0 0 1 2 3 4 4 4
  spline S129 degree 2 poles (1.0808, 5.6589) (1.1232, 5.6589) (1.2129, 5.7338) (1.2671, 5.8195) knots 0 0 0 1 2 2 2
  line L158 (1.2671, 5.8195) -> (1.2671, 6.3607)
  line L159 (1.2671, 6.3607) -> (1.4623, 6.3607)
  line L160 (1.4623, 6.3607) -> (1.4623, 5.5051)
  line L161 (1.4623, 5.5051) -> (1.2898, 5.5051)
  line L162 (1.2898, 5.5051) -> (1.2819, 5.6303)
  spline S130 degree 2 poles (1.2819, 5.6303) (1.2632, 5.5968) (1.2139, 5.5445) (1.1528, 5.5071) (1.0798, 5.4874) (1.0355, 5.4874) knots 0 0 0 1 2 3 4 4 4
  spline S131 degree 2 poles (1.0355, 5.4874) (0.9753, 5.4874) (0.8827, 5.5317) (0.8186, 5.6195) (0.7881, 5.7515) (0.791, 5.8383) knots 0 0 0 1 2 3 4 4 4
  line L163 (0.791, 5.8383) -> (0.9822, 5.8383)
  line L164 (0.1149, 6.3607) -> (0.1198, 6.2483)
  spline S132 degree 2 poles (0.1198, 6.2483) (0.1444, 6.2769) (0.1996, 6.3252) (0.2647, 6.3607) (0.3425, 6.3804) (0.3889, 6.3804) knots 0 0 0 1 2 3 4 4 4
  spline S133 degree 2 poles (0.3889, 6.3804) (0.45, 6.3804) (0.5416, 6.341) (0.6047, 6.272) (0.6363, 6.1744) (0.6363, 6.1152) knots 0 0 0 1 2 3 4 4 4
  spline S134 degree 2 poles (0.6363, 6.1152) (0.6363, 6.0551) (0.589, 5.9526) (0.4914, 5.8787) (0.3445, 5.8363) (0.2459, 5.8363) knots 0 0 0 1 2 3 4 4 4
  line L165 (0.2459, 5.8363) -> (0.1425, 5.8363)
  line L166 (0.1425, 5.8363) -> (0.1425, 5.785)
  spline S135 degree 2 poles (0.1425, 5.785) (0.1425, 5.7525) (0.1592, 5.6993) (0.1976, 5.6618) (0.2588, 5.6421) (0.3031, 5.6421) knots 0 0 0 1 2 3 4 4 4
  spline S136 degree 2 poles (0.3031, 5.6421) (0.3741, 5.6421) (0.5111, 5.6766) (0.5752, 5.7072) knots 0 0 0 1 2 2 2
  line L167 (0.5752, 5.7072) -> (0.5752, 5.5436)
  spline S137 degree 2 poles (0.5752, 5.5436) (0.518, 5.5189) (0.3682, 5.4874) (0.2873, 5.4874) knots 0 0 0 1 2 2 2
  spline S138 degree 2 poles (0.2873, 5.4874) (0.1996, 5.4874) (0.0725, 5.5229) (-0.0093, 5.5958) (-0.0488, 5.7042) (-0.0488, 5.7762) knots 0 0 0 1 2 3 4 4 4
  line L168 (-0.0488, 5.7762) -> (-0.0488, 6.3607)
  line L169 (-0.0488, 6.3607) -> (0.1149, 6.3607)
  line L170 (0.1425, 5.9832) -> (0.2588, 5.9832)
  spline S139 degree 2 poles (0.2588, 5.9832) (0.3071, 5.9832) (0.3741, 6.0029) (0.4165, 6.0384) (0.4362, 6.0847) (0.4362, 6.1103) knots 0 0 0 1 2 3 4 4 4
  spline S140 degree 2 poles (0.4362, 6.1103) (0.4362, 6.1626) (0.3741, 6.2178) (0.3199, 6.2178) knots 0 0 0 1 2 2 2
  spline S141 degree 2 poles (0.3199, 6.2178) (0.2795, 6.2178) (0.1937, 6.1557) (0.1425, 6.0975) knots 0 0 0 1 2 2 2
  line L171 (0.1425, 6.0975) -> (0.1425, 5.9832)
  line L172 (6.7863, 7.7935) -> (6.9055, 7.7935)
  line L173 (6.9055, 7.7935) -> (6.9234, 7.1698)
  line L174 (6.9234, 7.1698) -> (6.9314, 6.9306)
  line L175 (6.9314, 6.9306) -> (6.9736, 7.0695)
  line L176 (6.9736, 7.0695) -> (7.1062, 7.4673)
  line L177 (7.1062, 7.4673) -> (7.1904, 7.4673)
  line L178 (7.1904, 7.4673) -> (7.3176, 7.0847)
  line L179 (7.3176, 7.0847) -> (7.3598, 6.9306)
  line L180 (7.3598, 6.9306) -> (7.3624, 7.1806)
  line L181 (7.3624, 7.1806) -> (7.3777, 7.7935)
  line L182 (7.3777, 7.7935) -> (7.4933, 7.7935)
  line L183 (7.4933, 7.7935) -> (7.4494, 6.7935)
  line L184 (7.4494, 6.7935) -> (7.3042, 6.7935)
  line L185 (7.3042, 6.7935) -> (7.1832, 7.1698)
  line L186 (7.1832, 7.1698) -> (7.1438, 7.2971)
  line L187 (7.1438, 7.2971) -> (7.1062, 7.1698)
  line L188 (7.1062, 7.1698) -> (6.9789, 6.7935)
  line L189 (6.9789, 6.7935) -> (6.8293, 6.7935)
  line L190 (6.8293, 6.7935) -> (6.7863, 7.7935)
  line L191 (6.1985, 7.7935) -> (6.2012, 7.6905)
  spline S142 degree 2 poles (6.2012, 7.6905) (6.2576, 7.7523) (6.3741, 7.8069) (6.4377, 7.8069) knots 0 0 0 1 2 2 2
  spline S143 degree 2 poles (6.4377, 7.8069) (6.4969, 7.8069) (6.5811, 7.7738) (6.6348, 7.7146) (6.6608, 7.6349) (6.6608, 7.5883) knots 0 0 0 1 2 3 4 4 4
  spline S144 degree 2 poles (6.6608, 7.5883) (6.6608, 7.4727) (6.5058, 7.3419) (6.3544, 7.3419) knots 0 0 0 1 2 2 2
  line L192 (6.3544, 7.3419) -> (6.211, 7.3419)
  line L193 (6.211, 7.3419) -> (6.211, 7.2747)
  spline S145 degree 2 poles (6.211, 7.2747) (6.211, 7.2066) (6.2899, 7.125) (6.3705, 7.125) knots 0 0 0 1 2 2 2
  spline S146 degree 2 poles (6.3705, 7.125) (6.4288, 7.125) (6.5426, 7.1537) (6.6026, 7.1806) knots 0 0 0 1 2 2 2
  line L194 (6.6026, 7.1806) -> (6.6026, 7.0605)
  spline S147 degree 2 poles (6.6026, 7.0605) (6.5802, 7.0516) (6.5246, 7.0336) (6.4628, 7.0202) (6.3947, 7.0112) (6.3607, 7.0112) knots 0 0 0 1 2 3 4 4 4
  spline S148 degree 2 poles (6.3607, 7.0112) (6.2979, 7.0112) (6.1976, 7.0417) (6.1277, 7.1044) (6.0909, 7.1994) (6.0909, 7.2639) knots 0 0 0 1 2 3 4 4 4
  line L195 (6.0909, 7.2639) -> (6.0909, 7.7935)
  line L196 (6.0909, 7.7935) -> (6.1985, 7.7935)
  line L197 (6.211, 7.444) -> (6.3633, 7.444)
  spline S149 degree 2 poles (6.3633, 7.444) (6.4081, 7.444) (6.4727, 7.4638) (6.5139, 7.5005) (6.5345, 7.5516) (6.5345, 7.5838) knots 0 0 0 1 2 3 4 4 4
  spline S150 degree 2 poles (6.5345, 7.5838) (6.5345, 7.6062) (6.5219, 7.6465) (6.4942, 7.6779) (6.4503, 7.6967) (6.418, 7.6967) knots 0 0 0 1 2 3 4 4 4
  spline S151 degree 2 poles (6.418, 7.6967) (6.3768, 7.6967) (6.2702, 7.6403) (6.211, 7.5802) knots 0 0 0 1 2 2 2
  line L198 (6.211, 7.5802) -> (6.211, 7.444)
  spline S152 degree 2 poles (5.9019, 7.4252) (5.9019, 7.3276) (5.8544, 7.1752) (5.7648, 7.0704) (5.6402, 7.0157) (5.5641, 7.0157) knots 0 0 0 1 2 3 4 4 4
  spline S153 degree 2 poles (5.5641, 7.0157) (5.5309, 7.0157) (5.4673, 7.0256) (5.4359, 7.0354) knots 0 0 0 1 2 2 2
  line L199 (5.4359, 7.0354) -> (5.4359, 6.712)
  line L200 (5.4359, 6.712) -> (5.3159, 6.712)
  line L201 (5.3159, 6.712) -> (5.3159, 7.7935)
  line L202 (5.3159, 7.7935) -> (5.4234, 7.7935)
  line L203 (5.4234, 7.7935) -> (5.427, 7.6483)
  spline S154 degree 2 poles (5.427, 7.6483) (5.4771, 7.729) (5.5945, 7.8069) (5.6626, 7.8069) knots 0 0 0 1 2 2 2
  spline S155 degree 2 poles (5.6626, 7.8069) (5.7218, 7.8069) (5.8123, 7.7523) (5.8714, 7.6519) (5.9019, 7.5112) (5.9019, 7.4252) knots 0 0 0 1 2 3 4 4 4
  spline S156 degree 2 poles (5.78, 7.4172) (5.78, 7.556) (5.7056, 7.6931) (5.6384, 7.6931) knots 0 0 0 1 2 2 2
  spline S157 degree 2 poles (5.6384, 7.6931) (5.5927, 7.6931) (5.4924, 7.6026) (5.4359, 7.5139) knots 0 0 0 1 2 2 2
  line L204 (5.4359, 7.5139) -> (5.4359, 7.1573)
  spline S158 degree 2 poles (5.4359, 7.1573) (5.4655, 7.1421) (5.5372, 7.1259) (5.5721, 7.1259) knots 0 0 0 1 2 2 2
  spline S159 degree 2 poles (5.5721, 7.1259) (5.6698, 7.1259) (5.78, 7.2666) (5.78, 7.4172) knots 0 0 0 1 2 2 2
  spline S160 degree 2 poles (4.5085, 7.3688) (4.5085, 7.3974) (4.5094, 7.4351) (4.5112, 7.4521) knots 0 0 0 1 2 2 2
  line L205 (4.5112, 7.4521) -> (4.996, 7.4521)
  spline S161 degree 2 poles (4.996, 7.4521) (4.996, 7.5704) (4.8777, 7.6967) (4.7666, 7.6967) knots 0 0 0 1 2 2 2
  spline S162 degree 2 poles (4.7666, 7.6967) (4.7361, 7.6967) (4.6752, 7.6914) (4.6187, 7.6815) (4.5676, 7.6698) (4.5452, 7.6636) knots 0 0 0 1 2 3 4 4 4
  line L206 (4.5452, 7.6636) -> (4.5452, 7.7729)
  spline S163 degree 2 poles (4.5452, 7.7729) (4.5945, 7.7881) (4.7173, 7.8069) (4.7836, 7.8069) knots 0 0 0 1 2 2 2
  spline S164 degree 2 poles (4.7836, 7.8069) (4.8723, 7.8069) (5.0004, 7.7541) (5.082, 7.6519) (5.1214, 7.5041) (5.1214, 7.4109) knots 0 0 0 1 2 3 4 4 4
  spline S165 degree 2 poles (5.1214, 7.4109) (5.1214, 7.3293) (5.0793, 7.1851) (4.9986, 7.0758) (4.8822, 7.0112) (4.8078, 7.0112) knots 0 0 0 1 2 3 4 4 4
  spline S166 degree 2 poles (4.8078, 7.0112) (4.7352, 7.0112) (4.6241, 7.0623) (4.5479, 7.1546) (4.5085, 7.2872) (4.5085, 7.3688) knots 0 0 0 1 2 3 4 4 4
  spline S167 degree 2 poles (4.6331, 7.35) (4.6304, 7.298) (4.6528, 7.2138) (4.6994, 7.1519) (4.7675, 7.1179) (4.8132, 7.1179) knots 0 0 0 1 2 3 4 4 4
  spline S168 degree 2 poles (4.8132, 7.1179) (4.8526, 7.1179) (4.9171, 7.151) (4.9637, 7.2129) (4.9924, 7.298) (4.996, 7.35) knots 0 0 0 1 2 3 4 4 4
  line L207 (4.996, 7.35) -> (4.6331, 7.35)
  line L208 (3.306, 7.1358) -> (3.5112, 7.1358)
  line L209 (3.5112, 7.1358) -> (3.5112, 7.0256)
  line L210 (3.5112, 7.0256) -> (3.185, 7.0256)
  line L211 (3.185, 7.0256) -> (3.185, 7.6824)
  line L212 (3.185, 7.6824) -> (2.9798, 7.6824)
  line L213 (2.9798, 7.6824) -> (2.9798, 7.7935)
  line L214 (2.9798, 7.7935) -> (3.5336, 7.7935)
  line L215 (3.5336, 7.7935) -> (3.5336, 7.6824)
  line L216 (3.5336, 7.6824) -> (3.306, 7.6824)
  line L217 (3.306, 7.6824) -> (3.306, 7.1358)
  spline S169 degree 2 poles (3.2648, 6.703) (3.2442, 6.703) (3.2101, 6.7191) (3.1841, 6.7478) (3.1698, 6.7854) (3.1698, 6.8078) knots 0 0 0 1 2 3 4 4 4
  spline S170 degree 2 poles (3.1698, 6.8078) (3.1698, 6.8293) (3.1841, 6.8679) (3.2101, 6.8965) (3.2442, 6.9127) (3.2648, 6.9127) knots 0 0 0 1 2 3 4 4 4
  spline S171 degree 2 poles (3.2648, 6.9127) (3.2845, 6.9127) (3.3185, 6.8965) (3.3445, 6.8679) (3.3589, 6.8293) (3.3589, 6.8078) knots 0 0 0 1 2 3 4 4 4
  spline S172 degree 2 poles (3.3589, 6.8078) (3.3589, 6.7854) (3.3445, 6.7478) (3.3185, 6.7191) (3.2845, 6.703) (3.2648, 6.703) knots 0 0 0 1 2 3 4 4 4
  line L218 (2.7666, 7.0256) -> (2.6599, 7.0256)
  line L219 (2.6599, 7.0256) -> (2.6555, 7.1492)
  spline S173 degree 2 poles (2.6555, 7.1492) (2.625, 7.1098) (2.5685, 7.0569) (2.5139, 7.0247) (2.4574, 7.0112) (2.427, 7.0112) knots 0 0 0 1 2 3 4 4 4
  spline S174 degree 2 poles (2.427, 7.0112) (2.3203, 7.0112) (2.211, 7.151) (2.211, 7.2926) knots 0 0 0 1 2 2 2
  line L220 (2.211, 7.2926) -> (2.211, 7.7935)
  line L221 (2.211, 7.7935) -> (2.3311, 7.7935)
  line L222 (2.3311, 7.7935) -> (2.3311, 7.3034)
  spline S175 degree 2 poles (2.3311, 7.3034) (2.3311, 7.2129) (2.392, 7.1259) (2.4512, 7.1259) knots 0 0 0 1 2 2 2
  spline S176 degree 2 poles (2.4512, 7.1259) (2.4736, 7.1259) (2.5157, 7.1412) (2.5605, 7.177) (2.6142, 7.2379) (2.6465, 7.2836) knots 0 0 0 1 2 3 4 4 4
  line L223 (2.6465, 7.2836) -> (2.6465, 7.7935)
  line L224 (2.6465, 7.7935) -> (2.7666, 7.7935)
  line L225 (2.7666, 7.7935) -> (2.7666, 7.0256)
  spline S177 degree 2 poles (0.6277, 7.0991) (0.6277, 7.1609) (0.6689, 7.281) (0.7549, 7.3759) (0.8902, 7.4342) (0.9834, 7.4342) knots 0 0 0 1 2 3 4 4 4
  line L226 (0.9834, 7.4342) -> (1.0954, 7.4342)
  line L227 (1.0954, 7.4342) -> (1.0954, 7.7935)
  line L228 (1.0954, 7.7935) -> (1.2182, 7.7935)
  line L229 (1.2182, 7.7935) -> (1.2182, 6.7935)
  line L230 (1.2182, 6.7935) -> (0.9646, 6.7935)
  spline S178 degree 2 poles (0.9646, 6.7935) (0.8974, 6.7935) (0.7755, 6.8267) (0.6823, 6.9001) (0.6277, 7.0157) (0.6277, 7.0991) knots 0 0 0 1 2 3 4 4 4
  spline S179 degree 2 poles (0.7549, 7.1053) (0.7549, 7.0095) (0.8678, 6.9064) (0.97, 6.9064) knots 0 0 0 1 2 2 2
  line L231 (0.97, 6.9064) -> (1.0954, 6.9064)
  line L232 (1.0954, 6.9064) -> (1.0954, 7.3186)
  line L233 (1.0954, 7.3186) -> (0.9807, 7.3186)
  spline S180 degree 2 poles (0.9807, 7.3186) (0.8723, 7.3186) (0.7549, 7.2129) (0.7549, 7.1053) knots 0 0 0 1 2 2 2
  line L234 (-0.1716, 7.7935) -> (-0.0336, 7.7935)
  line L235 (-0.0336, 7.7935) -> (0.1008, 7.4736)
  spline S181 degree 2 poles (0.1008, 7.4736) (0.116, 7.4369) (0.1474, 7.3885) (0.1841, 7.3607) (0.2271, 7.3482) (0.254, 7.3482) knots 0 0 0 1 2 3 4 4 4
  line L236 (0.254, 7.3482) -> (0.3123, 7.3482)
  line L237 (0.3123, 7.3482) -> (0.3123, 7.7935)
  line L238 (0.3123, 7.7935) -> (0.4341, 7.7935)
  line L239 (0.4341, 7.7935) -> (0.4341, 6.7935)
  line L240 (0.4341, 6.7935) -> (0.194, 6.7935)
  spline S182 degree 2 poles (0.194, 6.7935) (0.1151, 6.7935) (0.0022, 6.832) (-0.0703, 6.9001) (-0.1035, 6.9978) (-0.1035, 7.0569) knots 0 0 0 1 2 3 4 4 4
  spline S183 degree 2 poles (-0.1035, 7.0569) (-0.1035, 7.1035) (-0.0793, 7.1869) (-0.03, 7.255) (0.0426, 7.3043) (0.0891, 7.3168) knots 0 0 0 1 2 3 4 4 4
  spline S184 degree 2 poles (0.0891, 7.3168) (0.0515, 7.3311) (-0.0022, 7.4037) (-0.0291, 7.4646) knots 0 0 0 1 2 2 2
  line L241 (-0.0291, 7.4646) -> (-0.1716, 7.7935)
  spline S185 degree 2 poles (0.0246, 7.0677) (0.0246, 6.9879) (0.1142, 6.9082) (0.1967, 6.9082) knots 0 0 0 1 2 2 2
  line L242 (0.1967, 6.9082) -> (0.3123, 6.9082)
  line L243 (0.3123, 6.9082) -> (0.3123, 7.2388)
  line L244 (0.3123, 7.2388) -> (0.2128, 7.2388)
  spline S186 degree 2 poles (0.2128, 7.2388) (0.1698, 7.2388) (0.0999, 7.2164) (0.0515, 7.1725) (0.0246, 7.1098) (0.0246, 7.0677) knots 0 0 0 1 2 3 4 4 4
  spline S187 degree 2 poles (-0.9082, 7.7559) (-0.8006, 7.806) (-0.6824, 7.806) knots 0 0 0 1 1 1
  spline S188 degree 2 poles (-0.6824, 7.806) (-0.4915, 7.806) (-0.2872, 7.5525) (-0.2872, 7.3043) knots 0 0 0 1 2 2 2
  spline S189 degree 2 poles (-0.2872, 7.3043) (-0.2872, 7.1842) (-0.3436, 6.9897) (-0.4476, 6.8544) (-0.5963, 6.781) (-0.6886, 6.781) knots 0 0 0 1 2 3 4 4 4
  spline S190 degree 2 poles (-0.6886, 6.781) (-0.7514, 6.781) (-0.8589, 6.8052) (-0.9082, 6.8293) knots 0 0 0 1 2 2 2
  line L245 (-0.9082, 6.8293) -> (-0.9082, 6.9629)
  spline S191 degree 2 poles (-0.9082, 6.9629) (-0.8598, 6.9333) (-0.7549, 6.9019) (-0.6931, 6.9019) knots 0 0 0 1 2 2 2
  spline S192 degree 2 poles (-0.6931, 6.9019) (-0.6295, 6.9019) (-0.5273, 6.9548) (-0.4557, 7.0552) (-0.4171, 7.1994) (-0.4171, 7.2926) knots 0 0 0 1 2 3 4 4 4
  spline S193 degree 2 poles (-0.4171, 7.2926) (-0.4171, 7.4871) (-0.5587, 7.6842) (-0.6958, 7.6842) knots 0 0 0 1 2 2 2
  spline S194 degree 2 poles (-0.6958, 7.6842) (-0.7531, 7.6842) (-0.8598, 7.6546) (-0.9082, 7.6277) knots 0 0 0 1 2 2 2
  line L246 (-0.9082, 7.6277) -> (-0.9082, 7.7559)
  point P0 (0, 0)
  dimension "d0" = 23.862
  dimension "d1" = 25
  dimension "d7" = 2
  dimension "d8" = 2
  dimension "d11" = 12.5
  dimension "d14" = 21
  dimension "d26" = 2
  constraints: 10 other
extrude "TEXTS_EXT" add sketch "text_front" along normal blind 0.03 separate body
sketch "REF_CON" plane through (0, 0, 1) normal (0, 0, 1) x (1, 0, 0)
  line L0 (-1.6061, 4.1358) -> (6.8939, 4.1358)
  line L1 (6.8939, 4.1358) -> (6.8939, -4.3642)
  line L2 (6.8939, -4.3642) -> (-1.6061, -4.3642)
  line L3 (-1.6061, -4.3642) -> (-1.6061, 4.1358)
  line L4 (-8.8261, -12.6142) -> (1.808, -12.6142) projected
  line L5 (12.1059, -10.6142) -> (12.1059, 10.3858) projected
  line L6 (3.6856, -12.6142) -> (10.1059, -12.6142) projected
  line L7 (12.1059, -10.6142) -> (12.1059, 10.3858) projected
  line L8 (-11.7561, 9.4548) -> (-11.7561, -9.6889) projected
  line L9 (-8.0373, -5.5033) -> (-5.9977, -5.5033)
  line L10 (-5.9977, -5.5033) -> (-5.9977, 2.9967)
  line L11 (-5.9977, 2.9967) -> (-8.1977, 2.9967)
  line L12 (-8.1977, 2.9967) -> (-8.0373, -5.5033)
  line L13 (-8.0373, -5.5033) -> (-5.9977, 2.9967) construction
  line L14 (-5.9977, -5.5033) -> (-8.1977, 2.9967) construction
  line L15 (-5.1142, -6.0033) -> (-9.2004, -6.0033)
  line L16 (-9.2004, -6.0033) -> (-9.2004, 3.175)
  line L17 (-9.2004, 3.175) -> (-5.1142, 3.175)
  line L18 (-5.1142, 3.175) -> (-5.1142, -6.0033)
  line L19 (1.8204, 12.3858) -> (-8.8385, 12.3858) projected
  point P0 (0, 0)
  point P1 (-7.0561, -1.4142)
  dimension "d74" = 8.5
  dimension "d75" = 8.5
  dimension "d78" = 5.212
  dimension "d79" = 8.25
  dimension "d82" = 4.7
  dimension "d86" = 2.2
  dimension "d87" = 8.5
  dimension "d88" = 0.5
  dimension "d98" = 13.8
  constraints: 28 end point, 3 perpendicular, 2 horizontal, 2 parallel, 2 point on line
  measures "d74" distance of L1.end L2.end
  measures "d75" distance of L0.end L1.end
  measures "d78" distance between parallel lines of L5 L1
  measures "d79" distance between parallel lines of L6 L2
  measures "d82" distance from line of L8 point (-7.056, -1.414)
  measures "d86" distance of L11.end L10.end
  measures "d87" distance of L10.end L9.end
  measures "d88" distance between parallel lines of L9 L15
  measures "d98" distance from line of L19 point (-7.056, -1.414)
extrude "CONN" add sketch "REF_CON" along normal blind 1 separate body contours L12 L11 L10 L9
extrude "CAM_BED" add sketch "REF_CON" along normal blind 0.1 separate body contours L0 L1 L2 L3
ref_plane "PLANO_CON" through (-5.9977, 2.9967, 2) normal (0, 0, -1) x (-1, 0, 0)
sketch "Boceto8" plane through (-5.9977, 2.9967, 2) normal (0, 0, -1) x (-1, 0, 0)
  line L0 (-0.8835, 0.1783) -> (-0.8835, -9) projected
  line L1 (3.2027, -9) -> (3.2027, 0.1783) projected
  line L2 (3.2027, 0.1783) -> (-0.8835, 0.1783) projected
  line L3 (-0.8835, -9) -> (3.2027, -9) projected
  point P0 (-5.9977, -2.9967)
extrude "CONN_TOP" add sketch "Boceto8" against normal blind 0.1 separate body
fillet "Empalme2" radius 0.2 4 edges at (-5.1142, 3.175, 2.05) (-9.2004, 3.175, 2.05) (-9.2004, -6.0033, 2.05) (-5.1142, -6.0033, 2.05)
sketch "REF_PADS_DRAW" plane through (0, 0, 1) normal (0, 0, 1) x (1, 0, 0)
  circle A0 centre (8.3476, 9.4204) radius 1.3903
  circle A1 centre (-5.5777, -10.1982) radius 1.4162
  circle A2 centre (-5.5777, -10.1982) radius 0.722
  circle A3 centre (8.3476, 9.4204) radius 0.7102
  point P0 (0, 0)
  constraints: 4 centre point, 2 coincident